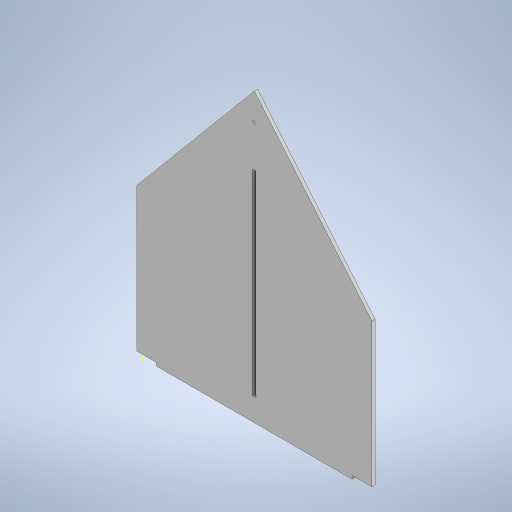
# Autodesk Inventor part: side
Saved by Autodesk Inventor 2023 (Build 270158000, 158)
## iProperties
Created: 2023-10-15
Part Number: side
Material: Generic
Document SubType Name: Modeling
Designer: Nate
Density: 1 g/cm^3
Appearance: Default
Author: Nate
Autodesk Inventor part; units mm, degrees
ref_plane "YZ Plane" through (0, 0, 0) normal (1, 0, 0) x (0, 1, 0)
ref_plane "XZ Plane" through (0, 0, 0) normal (0, 1, 0) x (-1, 0, 0)
ref_plane "XY Plane" through (0, 0, 0) normal (0, 0, 1) x (1, 0, 0)
sketch "Sketch1" plane through (0, 0, 0) normal (0, 0, 1) x (1, 0, 0)
  line L0 (0, 0) -> (-6.35, 0)
  line L1 (-6.35, 0) -> (-6.35, 381)
  line L2 (-6.35, 381) -> (0, 381)
  line L3 (0, 381) -> (0, 0)
  line L4 (-6.35, -38.1) -> (-558.8, -38.1)
  line L5 (-558.8, -38.1) -> (-558.8, 419.1)
  line L6 (-558.8, 419.1) -> (-6.35, 419.1)
  line L7 (-6.35, 419.1) -> (-6.35, -38.1)
  line L8 (-558.8, 190.5) -> (-285.75, -38.1)
  line L9 (-558.8, 190.5) -> (-285.75, 419.1)
  circle A0 centre (-506.349, 190.5) radius 3.175
  line L10 (-44.45, 187.325) -> (-425.45, 187.325)
  line L11 (-425.45, 187.325) -> (-425.45, 193.675)
  line L12 (-425.45, 193.675) -> (-44.45, 193.675)
  line L13 (-44.45, 193.675) -> (-44.45, 187.325)
  point P0 (-3.175, 0)
  point P1 (-44.45, 190.5)
  dimension "d0" = 6.35
  dimension "d1" = 381
  dimension "d2" = 552.45
  dimension "d3" = 457.2
  dimension "d4" = 38.1
  dimension "d5" = 228.6
  dimension "d6" = 279.4
  dimension "d7" = 228.6
  dimension "d9" = 6.35
  dimension "d10" = 228.6
  dimension "d11" = 499.999
  dimension "d12" = 279.4
  dimension "d15" = 381
  dimension "d16" = 6.35
  dimension "d17" = 225.425
  dimension "d18" = 38.1
  constraints: 28 end point, 6 parallel, 3 horizontal, 3 midpoint, 3 perpendicular, 3 point on line, 1 centre point
  measures "d0" distance of L1.end L2.end
  measures "d1" distance of L0.end L1.end
  measures "d2" distance of L5.end L6.end
  measures "d3" distance between parallel lines of L6 L4
  measures "d4" distance from line of L4 point (-3.175, 0)
  measures "d5" distance from line of L8.start L4
  measures "d6" distance from line of L1 L8.end
  measures "d7" distance from line of L6 L8.start
  measures "d9" diameter of A0
  measures "d10" distance from line of L6 A0.centre
  measures "d11" distance from line of L1 A0.centre
  measures "d12" distance from line of L7 L9.end
  measures "d15" distance of L11.end L12.end
  measures "d16" distance between parallel lines of L12 L10
  measures "d17" distance between parallel lines of L10 L4
  measures "d18" distance from line of point (-44.45, 190.5) L7
extrude "Extrusion1" add sketch "Sketch1" along normal blind 6.35 contours L0 L1 L2 L3 | L7 L4 L8 L9 L6 L1
sketch "Sketch2" plane through (0, 0, 6.35) normal (0, 0, 1) x (1, 0, 0)
  point P0 (0, 0)
move or copy body "Move Body1" bodies to move or copy 1 copy no rotation origin (0, 0, 0) rotation axis (0, 0, 1) rotation angle -90
move or copy body "Move Body2" bodies to move or copy 1 copy no translate (25.4, 0, 0)
body "Solid1"
